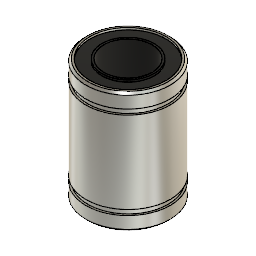
LM12UU_F01 (Autodesk Fusion 360 design; units mm, degrees)
Autodesk Fusion 360 part; units mm, degrees
sketch "スケッチ1" plane through (0, 0, 0) normal (0, 1, 0) x (1, 0, 0)
  line L0 (0, 0) -> (0, -15)
  line L1 (0, -15) -> (10.5, -15)
  line L2 (10.5, -15) -> (10.5, -11.5)
  line L3 (10.5, -11.5) -> (10, -11.5)
  line L4 (10, -11.5) -> (10, -10.2)
  line L5 (10, -10.2) -> (10.5, -10.2)
  line L6 (10.5, -10.2) -> (10.5, 10.2)
  line L7 (10.5, 10.2) -> (10, 10.2)
  line L8 (10, 10.2) -> (10, 11.5)
  line L9 (10, 11.5) -> (10.5, 11.5)
  line L10 (10.5, 11.5) -> (10.5, 15)
  line L11 (10.5, 15) -> (0, 15)
  line L12 (0, 15) -> (0, 0)
  line L13 (9.5, -15) -> (9.5, 15)
  line L14 (6.5, -15) -> (6.5, -14.5)
  line L15 (6.5, -14.5) -> (9.5, -14.5)
  line L16 (6, -15) -> (6, 15)
  line L17 (6.5, 15) -> (6.5, 14.5)
  line L18 (6.5, 14.5) -> (9.5, 14.5)
  dimension "d1" = 10.5
  dimension "d2" = 15
  dimension "d3" = 15
  dimension "d4" = 10
  dimension "d5" = 3.5
  dimension "d6" = 1.3
  dimension "d7" = 3.5
  dimension "d8" = 1.3
  dimension "d9" = 9.5
  dimension "d10" = 6
  dimension "d11" = 0.5
  dimension "d12" = 0.5
  dimension "d13" = 0.5
  measures "d1" distance of L0 L2
  measures "d2" distance of L0.start L1
  measures "d3" distance of L0.start L11
  measures "d4" distance of L0 L4
  measures "d5" distance of L1 L3
  measures "d9" distance of L0 L13
  measures "d10" distance of L0 L16
  measures "d11" distance of L14 L16
revolve "回転1" add sketch "スケッチ1" angle 360 about axis through (0, 0, 0) along (0, 0, 1) contours L1 L11 L13 L14 L15 L16 L17 L18 makes body 1
revolve "回転2" add sketch "スケッチ1" angle 360 about axis through (0, 0, 1.75) along (0, 0, 1) separate body contours L1 L2 L3 L4 L5 L6 L7 L8 L9 L10 L11 L13 makes body 2
chamfer "面取り1" distance 0.5 angle 45 2 edges at (-9.7894, -3.797, 15) (-9.7894, -3.797, -15) on bodies 2
equation "d3 = d2"
equation "d7 = d5"
equation "d8 = d6"
equation "d13 = d12"
